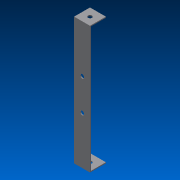
# Autodesk Inventor part: SupportBAr
Saved by Autodesk Inventor 2013 (Build 170138000, 138)
## iProperties
Created: 2013-07-15
Part Number: SupportBAr
Material: Aluminum 6061
Document SubType Name: Modeling
Designer: root
Density: 1 g/cm^3
Author: root
Autodesk Inventor part; units mm, degrees
ref_plane "YZ Plane" through (0, 0, 0) normal (1, 0, 0) x (0, 1, 0)
ref_plane "XZ Plane" through (0, 0, 0) normal (0, 1, 0) x (-1, 0, 0)
ref_plane "XY Plane" through (0, 0, 0) normal (0, 0, 1) x (1, 0, 0)
sketch "Sketch1" plane through (0, 0, 0) normal (1, 0, 0) x (0, 1, 0)
  line L0 (0, 0) -> (0, 25.4)
  line L1 (0, 25.4) -> (203.2, 25.4)
  line L2 (203.2, 25.4) -> (203.2, 0)
  line L3 (203.2, 0) -> (201.6125, 0)
  line L4 (201.6125, 0) -> (201.6125, 23.8125)
  line L5 (201.6125, 23.8125) -> (1.5875, 23.8125)
  line L6 (1.5875, 23.8125) -> (1.5875, 0)
  line L7 (1.5875, 0) -> (0, 0)
  dimension "d0" = 25.4
  dimension "d1" = 203.2
  dimension "d2" = 1.5875
  dimension "d3" = 1.5875
  dimension "d4" = 1.5875
  dimension "d5" = 25.4
  constraints: 16 end point, 6 parallel, 1 perpendicular, 1 vertical
  measures "d0" distance of L0.start L0.end
  measures "d1" distance of L0.end L1.end
  measures "d2" distance between parallel lines of L5 L1
  measures "d3" distance of L6.end L0.start
  measures "d4" distance of L2.end L3.end
  measures "d5" distance of L1.end L2.end
extrude "Extrusion1" add sketch "Sketch1" along normal blind 25.4
sketch "Sketch2" plane through (0, 203.2, 25.4) normal (0, 1, 0) x (1, 0, 0)
  line L0 (25.4, 25.4) -> (25.4, 0) projected
  line L1 (0, 25.4) -> (25.4, 25.4) projected
  point P0 (12.7, 12.7)
  dimension "d8" = 12.7
  dimension "d9" = 12.7
  measures "d8" distance from line of point (12.7, 12.7) L0
  measures "d9" distance from line of point (12.7, 12.7) L1
hole "Hole1" at (12.7, 203.2, 12.7) direction (0, -1, 0) diameter 6.35 end through all
sketch "Sketch3" plane through (0, 0, 25.4) normal (0, 0, 1) x (1, 0, 0)
  line L0 (0, 0) -> (0, 203.2) projected
  line L1 (0, 0) -> (25.4, 0) projected
  line L2 (25.4, 203.2) -> (25.4, 0) projected
  line L3 (0, 101.6) -> (25.4, 101.6)
  point P0 (12.7, 127)
  point P1 (12.7, 76.2)
  dimension "d17" = 12.7
  dimension "d18" = 12.7
  dimension "d28" = 101.6
  dimension "d29" = 50.8
  dimension "d30" = 25.4
  constraints: 2 end point, 2 midpoint, 1 perpendicular
  measures "d17" distance from line of point (12.7, 76.2) L2
  measures "d18" distance from line of point (12.7, 127) L0
  measures "d28" distance between parallel lines of L1 L3
  measures "d29" distance of point (12.7, 127) point (12.7, 76.2)
  measures "d30" distance from line of point (12.7, 127) L3
hole "Hole2" at (12.7, 127, 25.4) at (12.7, 76.2, 25.4) direction (0, 0, -1) diameter 6.35 end through all
body "Solid1"
